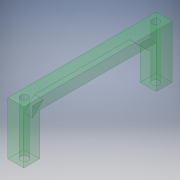
# Autodesk Inventor part: SparkMaxTop
Saved by Autodesk Inventor 2019 (Build 230136000, 136)
## iProperties
Created: 2019-12-12
Part Number: SparkMaxTop
Material: Generic
Document SubType Name: Modeling
Designer: james
Density: 1 g/cm^3
Appearance: Clear - Green 1
Mass: 6.14515 g
Surface Area: 39.516 cm^2
Volume: 6.14515 cm^3
Author: james
Autodesk Inventor part; units mm, degrees
ref_plane "YZ Plane" through (0, 0, 0) normal (1, 0, 0) x (0, 1, 0)
ref_plane "XZ Plane" through (0, 0, 0) normal (0, 1, 0) x (-1, 0, 0)
ref_plane "XY Plane" through (0, 0, 0) normal (0, 0, 1) x (1, 0, 0)
sketch "Sketch1" plane through (0, 0, 0) normal (1, 0, 0) x (0, 1, 0)
  line L0 (22.0204, 54.3207) -> (-9.7296, 54.3207)
  line L1 (-9.7296, -34.5793) -> (22.0204, -34.5793)
  line L2 (22.0204, -34.5793) -> (22.0204, 54.3207)
  line L3 (15.6704, 44.7957) -> (-9.7296, 44.7957)
  line L4 (-9.7296, -25.0543) -> (15.6704, -25.0543)
  line L5 (15.6704, -25.0543) -> (15.6704, 44.7957)
  line L6 (-9.7296, 54.3207) -> (-9.7296, 44.7957)
  line L7 (-9.7296, -25.0543) -> (-9.7296, -34.5793)
  dimension "d0" = 88.9
  dimension "d2" = 6.35
  dimension "d3" = 9.525
  dimension "d4" = 9.525
  dimension "d7" = 25.4
  dimension "d8" = 0
  constraints: 16 end point, 4 parallel, 2 horizontal, 2 perpendicular
  measures "d0" distance between parallel lines of L1 L0
  measures "d2" distance between parallel lines of L2 L5
  measures "d3" distance between parallel lines of L0 L3
  measures "d4" distance between parallel lines of L1 L4
  measures "d7" distance between parallel lines of L6 L5
  measures "d8" distance between parallel lines of L6 L7
extrude "Extrusion1" add sketch "Sketch1" along normal blind 9.525
sketch "Sketch2" plane through (0, 22.0204, 54.3207) normal (0, 1, 0) x (1, 0, 0)
  line L0 (0, 88.9) -> (9.525, 88.9) projected
  line L1 (0, 0) -> (9.525, 0) projected
  line L2 (0, 88.9) -> (0, 0) projected
  point P0 (0, 54.3207)
  point P1 (4.7625, 5.08)
  point P2 (4.7625, 83.82)
  dimension "d9" = 5.08
  dimension "d10" = 5.08
  dimension "d11" = 4.7625
  dimension "d12" = 0
  measures "d9" distance from line of L0 point (4.763, 83.82)
  measures "d10" distance from line of L1 point (4.763, 5.08)
  measures "d11" distance from line of L2 point (4.763, 5.08)
  measures "d12" horizontal distance of point (4.763, 5.08) point (4.763, 83.82)
hole "Hole1" at (4.7625, 22.0204, 49.2407) at (4.7625, 22.0204, -29.4993) direction (0, -1, 0) diameter 4.4958 end through all clearance for "Flat Head Machine Screw (82)" size "#8" standard "Ansi Unified Screw Threads"
sketch "Sketch4" plane through (0, 0, 0) normal (-1, 0, 0) x (0, 0, 1)
  line L0 (44.7957, 15.6704) -> (-25.0543, 15.6704) projected
  line L1 (44.7957, -9.7296) -> (44.7957, 15.6704) projected
  line L2 (-25.0543, 15.6704) -> (-25.0543, -9.7296) projected
  line L3 (-25.0543, 9.3204) -> (-18.7043, 15.6704)
  line L4 (-18.7043, 15.6704) -> (-25.0543, 15.6704)
  line L5 (-25.0543, 15.6704) -> (-25.0543, 9.3204)
  line L6 (44.7957, 9.3204) -> (44.7957, 15.6704)
  line L7 (44.7957, 15.6704) -> (38.4457, 15.6704)
  line L8 (38.4457, 15.6704) -> (44.7957, 9.3204)
  point P0 (0, 0)
  dimension "d20" = 45
  dimension "d21" = 6.35
  dimension "d22" = 0
  dimension "d23" = 0
  dimension "d24" = 45
  dimension "d25" = 6.35
  dimension "d26" = 0
  dimension "d27" = 0
  constraints: 12 end point, 2 perpendicular, 1 horizontal, 1 vertical
  measures "d20" angle of L4 L3
  measures "d21" distance of L4.end L3.start
  measures "d22" distance between parallel lines of L2 L5
  measures "d23" distance between parallel lines of L0 L4
  measures "d24" angle of L7 L8
  measures "d25" distance of L6.end L7.end
  measures "d26" distance between parallel lines of L0 L7
  measures "d27" distance between parallel lines of L1 L6
extrude "Extrusion2" add sketch "Sketch4" against normal blind 5.3
body "Solid1"
